Autodesk Fusion 360 part; units mm, degrees
note: some values were not read from the file. Chosen so that the rebuilt part matches the saved one: which bodies a step acts on.
(part 4 of 4)
equation "d695 = spinner_bar_W * 3"
named bodies: "Base_Plate_Al", "Left_Side_Plate_Al", "Right_Side_Plate_Al", "Left_Wheel", "Right_Wheel", "Top_Cover", "TT_Gearbox_L", "TT_Motor_Can_L", "TT_Gearbox_R", "TT_Motor_Can_R", "Battery_and_Tray", "Front_Wedge_L", "Front_Wedge_R", "Spinner_Shaft", "Left_Support", "Right_Support", "Spinner_Motor", "Standoff_1", "Standoff_2", "Standoff_3", "Standoff_4", "Battery_Holder", "Spinner_Motor_Cradle", "TT_Motor_Mount_L", "TT_Motor_Clamp_L", "TT_Motor_Mount_R", "TT_Motor_Clamp_R", "Batt_Post_1", "Batt_Post_2", "Batt_Post_3", "Batt_Post_4", "Disconnect_Post_1", "Disconnect_Post_2", "Rear_Panel", "Weapon_Pulley", "Motor_Pulley", "ESC_Tekko32", "Holder_ESC_Tekko32", "Rx_ER6", "Holder_Rx_ER6", "UBEC_5A", "Holder_UBEC_5A", "DRV8874_A", "Holder_DRV8874_A", "DRV8874_B", "Holder_DRV8874_B", "ESP32_DevKit", "ESP32_Module", "ESP32_Dupont_Keepout_A", "ESP32_Dupont_Keepout_B", "Holder_ESP32", "FingerTech_Switch_Adapter", "FingerTech_Mini_Switch_Envelope", "Spinner_Bar", "Spinner_Sweep_Envelope", "Lifter_Spatula_62mm", "Lifter_Hinge_Boss", "Lifter_Pivot_Support_L", "Lifter_Pivot_Support_R", "Lifter_Pivot_Pin_6mm", "Servo_30kgcm_Envelope_Only", "Lifter_Servo_Horn_Envelope_Only", "Lifter_Linkage_Envelope_Only", "Grabber_Upper_Jaw", "Grabber_Arm_L", "Grabber_Arm_R", "Grabber_Pivot_Pin_6mm", "Grabber_Pivot_Bracket_L", "Grabber_Pivot_Bracket_R", "Grabber_Second_Servo_Envelope_Only", "Grabber_Linkage_Envelope_Only", "Repeat_40kg_Servo_MaxEnvelope", "Lifter_Servo_Base_Rail_L", "Lifter_Servo_Base_Rail_R", "Lifter_Aluminium_Horn", "Lifter_Connecting_Rod", "Lifter_Lower_Hard_Stop", "BBB_22mm_Gearmotor_L", "BBB_4mm_Output_Shaft_L", "BBB_Face_Mount_26mm_L", "BBB_Motor_Cradle_L", "Repeat_4mm_Clamp_Hub_L", "BBB_22mm_Gearmotor_R", "BBB_4mm_Output_Shaft_R", "BBB_Face_Mount_26mm_R", "BBB_Motor_Cradle_R", "Repeat_4mm_Clamp_Hub_R", "BBB_Dual_Brushed_ESC_v2_Envelope", "Battery_Clamp_Bar_1", "Battery_Clamp_Bar_2", "Lifter_Servo_Clamp_Bar_L", "Lifter_Servo_Clamp_Post_L_Rear", "Lifter_Servo_Clamp_Post_L_Front", "Lifter_Servo_Clamp_Bar_R", "Lifter_Servo_Clamp_Post_R_Rear", "Lifter_Servo_Clamp_Post_R_Front", "Lifter_Pin_C_Clip_L", "Lifter_Pin_C_Clip_R"
